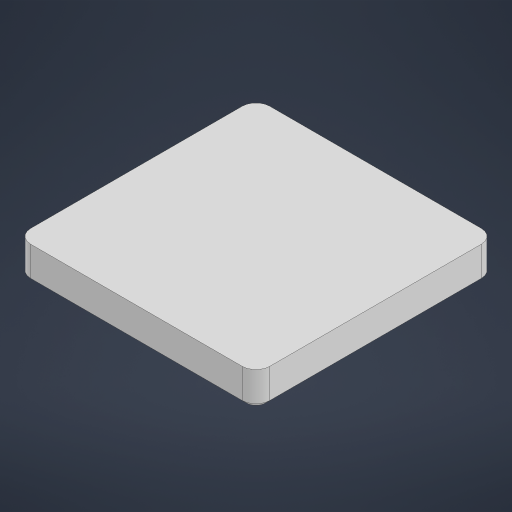
# Autodesk Inventor part: top_insert
Saved by Autodesk Inventor 2024 (Build 280153000, 153)
## iProperties
Created: 2024-03-20
Part Number: top_insert
Material: Všeobecné
Document SubType Name: Modeling
Designer: Simak
Density: 1 g/cm^3
Appearance: Výchozí
Author: Simak
Autodesk Inventor part; units mm, degrees
ref_plane "YZ Plane" through (0, 0, 0) normal (1, 0, 0) x (0, 1, 0)
ref_plane "XZ Plane" through (0, 0, 0) normal (0, 1, 0) x (-1, 0, 0)
ref_plane "XY Plane" through (0, 0, 0) normal (0, 0, 1) x (1, 0, 0)
sketch "Náčrt1" plane through (0, 0, 0) normal (0, 1, 0) x (-1, 0, 0)
  line L0 (52.5, 52.5) -> (-52.5, 52.5)
  line L1 (-52.5, 52.5) -> (-52.5, -52.5)
  line L2 (-52.5, -52.5) -> (52.5, -52.5)
  line L3 (52.5, -52.5) -> (52.5, 52.5)
  line L4 (52.5, 52.5) -> (0, 0) construction
  line L5 (0, 0) -> (52.5, -52.5) construction
  line L6 (0, 0) -> (-52.5, -52.5) construction
  dimension "d0" = 105
  constraints: 14 end point, 3 equal length, 2 parallel, 1 horizontal, 1 perpendicular
  measures "d0" distance of L1.end L2.end
extrude "Vysunutí1" add sketch "Náčrt1" along normal blind 15
fillet "Zaoblení1" radius 6 4 edges at (52.5, 7.5, 52.5) (-52.5, 7.5, 52.5) (52.5, 7.5, -52.5) (-52.5, 7.5, -52.5)
chamfer "Zkosení1" distance 2 angle 45 8 edges at (52.5, 0, 0) (50.7426, 0, -50.7426) (0, 0, -52.5) (-50.7426, 0, -50.7426) (-52.5, 0, 0) (-50.7426, 0, 50.7426) (0, 0, 52.5) (50.7426, 0, 50.7426)
